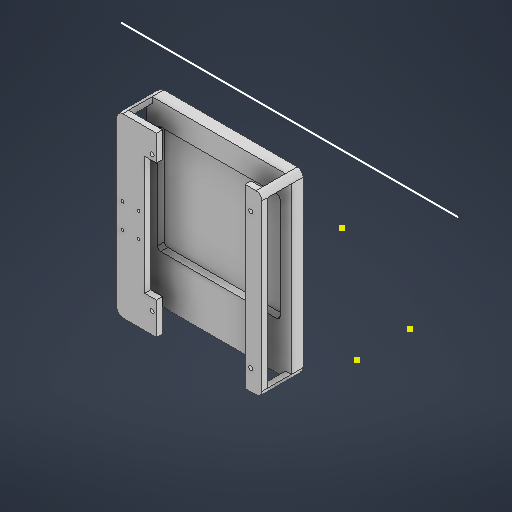
# Autodesk Inventor part: Box2
Saved by Autodesk Inventor 2026 (Build 300175000, 175)
## iProperties
Created: 2025-12-06
Part Number: Box2
Material: Generic
Document SubType Name: Modeling
Designer: sudis
Density: 1 g/cm^3
Appearance: Default
Author: sudis
Autodesk Inventor part; units mm, degrees
ref_plane "Work Plane1" through (-141.8656, 16.9601, -97.2578) normal (0, 0, -1) x (-1, 0, 0)
sketch "Sketch1" plane through (-141.8656, 16.9601, -97.2578) normal (0, 0, -1) x (-1, 0, 0)
  line L0 (61.5, 85.55) -> (-61.5, 85.55)
  line L1 (-61.5, 85.55) -> (-61.5, -85.55)
  line L2 (-61.5, -85.55) -> (61.5, -85.55)
  line L3 (61.5, -85.55) -> (61.5, 85.55)
  line L4 (-49.2, 45.05) -> (49.2, 45.05) projected
  arc A0 (-49.2, 45.25) -> (-51.5, 42.95) centre (-49.2, 42.95) ccw projected
  line L5 (-51.5, -42.95) -> (-51.5, 42.95) projected
  arc A1 (-51.5, -42.95) -> (-49.2, -45.25) centre (-49.2, -42.95) ccw projected
  line L6 (49.2, -45.25) -> (-49.2, -45.25) projected
  arc A2 (49.2, -45.25) -> (51.5, -42.95) centre (49.2, -42.95) ccw projected
  line L7 (51.5, 42.95) -> (51.5, -42.95) projected
  arc A3 (51.5, 42.95) -> (49.2, 45.25) centre (49.2, 42.95) ccw projected
  line L8 (-49.2, 45.25) -> (49.2, 45.25) projected
  line L9 (-1.4388, 35.9111) -> (-1.4388, 43.9889) projected
  ellipse E0 centre (-1.2387, 43.9887) end of major axis (-1.3802, 44.1302) minor radius 0.2 (-1.2389, 44.1888) -> (-1.4388, 43.9889) ccw projected
  line L10 (1.2389, 44.1888) -> (-1.2389, 44.1888) projected
  ellipse E1 centre (1.2387, 43.9887) end of major axis (1.3802, 44.1302) minor radius 0.2 (1.4388, 43.9889) -> (1.2389, 44.1888) ccw projected
  line L11 (1.4388, 43.9889) -> (1.4388, 35.9111) projected
  ellipse E2 centre (1.0386, 35.9114) end of major axis (1.3217, 35.6283) minor radius 0.4 (1.0389, 35.5112) -> (1.4388, 35.9111) ccw projected
  line L12 (-1.0389, 35.5112) -> (1.0389, 35.5112) projected
  ellipse E3 centre (-1.0386, 35.9114) end of major axis (-1.3217, 35.6283) minor radius 0.4 (-1.4388, 35.9111) -> (-1.0389, 35.5112) ccw projected
  arc A4 (1.3, 34.75) -> (1.9, 35.35) centre (1.3, 35.35) ccw projected
  line L13 (1.9, 40.81) -> (1.9, 35.35) projected
  arc A5 (2.1, 41.01) -> (1.9, 40.81) centre (2.1, 40.81) ccw projected
  line L14 (2.1, 41.01) -> (2.9, 41.01) projected
  arc A6 (2.9, 41.01) -> (2.9, 41.95) centre (2.9, 41.48) ccw projected
  line L15 (2.9, 41.95) -> (2.1, 41.95) projected
  arc A7 (1.9, 42.15) -> (2.1, 41.95) centre (2.1, 42.15) ccw projected
  line L16 (1.9, 43.9887) -> (1.9, 42.15) projected
  ellipse E4 centre (2.1, 43.9887) end of major axis (2.1, 44.1888) minor radius 0.2 (2.1, 44.1888) -> (1.9, 43.9887) ccw projected
  line L17 (48.7, 44.1888) -> (2.1, 44.1888) projected
  ellipse E5 centre (48.7, 43.1884) end of major axis (48.7, 44.1888) minor radius 1 (49.7, 43.1884) -> (48.7, 44.1888) ccw projected
  line L18 (49.7, 43.1884) -> (49.7, 39.02) projected
  arc A8 (49.5, 38.82) -> (49.7, 39.02) centre (49.5, 39.02) ccw projected
  line L19 (49.5, 38.82) -> (49.3, 38.82) projected
  arc A9 (49.3, 38.82) -> (49.3, 37.88) centre (49.3, 38.35) ccw projected
  line L20 (49.3, 37.88) -> (49.5, 37.88) projected
  arc A10 (49.7, 37.68) -> (49.5, 37.88) centre (49.5, 37.68) ccw projected
  line L21 (49.7, 37.68) -> (49.7, 33.65) projected
  arc A11 (48.7, 32.65) -> (49.7, 33.65) centre (48.7, 33.65) ccw projected
  line L22 (44.3574, 32.65) -> (48.7, 32.65) projected
  line L23 (44.3574, 32.65) -> (44.3574, 31.25) projected
  arc A12 (44.3574, 31.25) -> (46, 29.6074) centre (46, 31.25) ccw projected
  line L24 (46, 29.6074) -> (49.0579, 29.6074) projected
  spline S0 degree 3 poles (49.0579, 29.6074) (49.1602, 29.6074) (49.2528, 29.5891) (49.3382, 29.5567) (49.4237, 29.5242) (49.5019, 29.4774) (49.5659, 29.4253) (49.63, 29.3732) (49.6799, 29.3158) (49.7211, 29.2545) (49.7623, 29.1932) (49.7948, 29.128) (49.8186, 29.0541) (49.8423, 28.9803) (49.8574, 28.8977) (49.8574, 28.8079) knots 0.000001 0.000001 0.000001 0.000001 0.2 0.2 0.2 0.4 0.4 0.4 0.6 0.6 0.6 0.8 0.8 0.8 1 1 1 1 projected
  line L25 (49.8574, 28.8079) -> (49.8574, -24.3079) projected
  spline S1 degree 3 poles (49.8574, -24.3079) (49.8574, -24.3965) (49.8435, -24.4795) (49.8172, -24.5583) (49.7909, -24.6372) (49.7523, -24.712) (49.7048, -24.7778) (49.6573, -24.8437) (49.601, -24.9008) (49.5354, -24.9492) (49.4699, -24.9976) (49.3952, -25.0375) (49.3152, -25.0649) (49.2351, -25.0923) (49.1498, -25.1074) (49.0579, -25.1074) knots 0 0 0 0 0.2 0.2 0.2 0.4 0.4 0.4 0.6 0.6 0.6 0.8 0.8 0.8 1 1 1 1 projected
  line L26 (49.0579, -25.1074) -> (46, -25.1074) projected
  arc A13 (46, -25.1074) -> (46, -28.3926) centre (46, -26.75) ccw projected
  line L27 (46, -28.3926) -> (49.0579, -28.3926) projected
  spline S2 degree 3 poles (49.0579, -28.3926) (49.1602, -28.3926) (49.2528, -28.4109) (49.3382, -28.4433) (49.4237, -28.4758) (49.5019, -28.5226) (49.5659, -28.5747) (49.63, -28.6268) (49.6799, -28.6842) (49.7211, -28.7455) (49.7623, -28.8068) (49.7948, -28.872) (49.8186, -28.9459) (49.8423, -29.0197) (49.8574, -29.1023) (49.8574, -29.1921) knots 0.000001 0.000001 0.000001 0.000001 0.2 0.2 0.2 0.4 0.4 0.4 0.6 0.6 0.6 0.8 0.8 0.8 1 1 1 1 projected
  line L28 (49.8574, -29.1921) -> (49.8574, -42.95) projected
  arc A14 (49.2, -43.6074) -> (49.8574, -42.95) centre (49.2, -42.95) ccw projected
  line L29 (49.2, -43.6074) -> (-49.2, -43.6074) projected
  arc A15 (-49.8574, -42.95) -> (-49.2, -43.6074) centre (-49.2, -42.95) ccw projected
  line L30 (-49.8574, -42.95) -> (-49.8574, -29.1921) projected
  spline S3 degree 3 poles (-49.8574, -29.1921) (-49.8574, -29.1035) (-49.8435, -29.0205) (-49.8172, -28.9417) (-49.7909, -28.8628) (-49.7523, -28.788) (-49.7048, -28.7222) (-49.6573, -28.6563) (-49.601, -28.5992) (-49.5354, -28.5508) (-49.4699, -28.5024) (-49.3952, -28.4625) (-49.3152, -28.4351) (-49.2351, -28.4077) (-49.1498, -28.3926) (-49.0579, -28.3926) knots 0 0 0 0 0.2 0.2 0.2 0.4 0.4 0.4 0.6 0.6 0.6 0.8 0.8 0.8 1 1 1 1 projected
  line L31 (-49.0579, -28.3926) -> (-40, -28.3926) projected
  arc A16 (-40, -28.3926) -> (-40, -25.1074) centre (-40, -26.75) ccw projected
  line L32 (-40, -25.1074) -> (-49.0579, -25.1074) projected
  spline S4 degree 3 poles (-49.0579, -25.1074) (-49.1602, -25.1074) (-49.2528, -25.0891) (-49.3382, -25.0567) (-49.4237, -25.0242) (-49.5019, -24.9774) (-49.5659, -24.9253) (-49.63, -24.8732) (-49.6799, -24.8158) (-49.7211, -24.7545) (-49.7623, -24.6932) (-49.7948, -24.628) (-49.8186, -24.5541) (-49.8423, -24.4803) (-49.8574, -24.3977) (-49.8574, -24.3079) knots 0.000001 0.000001 0.000001 0.000001 0.2 0.2 0.2 0.4 0.4 0.4 0.6 0.6 0.6 0.8 0.8 0.8 1 1 1 1 projected
  line L33 (-49.8574, -24.3079) -> (-49.8574, 25.9079) projected
  spline S5 degree 3 poles (-49.8574, 25.9079) (-49.8574, 26.0102) (-49.8391, 26.1028) (-49.8067, 26.1882) (-49.7742, 26.2737) (-49.7274, 26.3519) (-49.6753, 26.4159) (-49.6232, 26.48) (-49.5658, 26.5299) (-49.5045, 26.5711) (-49.4432, 26.6123) (-49.378, 26.6448) (-49.3041, 26.6686) (-49.2303, 26.6923) (-49.1477, 26.7074) (-49.0579, 26.7074) knots 0.000001 0.000001 0.000001 0.000001 0.2 0.2 0.2 0.4 0.4 0.4 0.6 0.6 0.6 0.8 0.8 0.8 1 1 1 1 projected
  line L34 (-49.0579, 26.7074) -> (-36.4, 26.7074) projected
  arc A17 (-36.4, 26.7074) -> (-34.3574, 28.75) centre (-36.4, 28.75) ccw projected
  line L35 (-34.3574, 28.75) -> (-34.3574, 32.65) projected
  line L36 (-34.3574, 32.65) -> (-48.7, 32.65) projected
  arc A18 (-49.7, 33.65) -> (-48.7, 32.65) centre (-48.7, 33.65) ccw projected
  line L37 (-49.7, 33.65) -> (-49.7, 37.68) projected
  arc A19 (-49.5, 37.88) -> (-49.7, 37.68) centre (-49.5, 37.68) ccw projected
  line L38 (-49.5, 37.88) -> (-49.3, 37.88) projected
  arc A20 (-49.3, 37.88) -> (-49.3, 38.82) centre (-49.3, 38.35) ccw projected
  line L39 (-49.3, 38.82) -> (-49.5, 38.82) projected
  arc A21 (-49.7, 39.02) -> (-49.5, 38.82) centre (-49.5, 39.02) ccw projected
  line L40 (-49.7, 39.02) -> (-49.7, 43.1884) projected
  ellipse E6 centre (-48.7, 43.1884) end of major axis (-48.7, 44.1888) minor radius 1 (-48.7, 44.1888) -> (-49.7, 43.1884) ccw projected
  line L41 (-2.1, 44.1888) -> (-48.7, 44.1888) projected
  ellipse E7 centre (-2.1, 43.9887) end of major axis (-2.1, 44.1888) minor radius 0.2 (-1.9, 43.9887) -> (-2.1, 44.1888) ccw projected
  line L42 (-1.9, 35.69) -> (-1.9, 43.9887) projected
  line L43 (-1.9, 35.69) -> (-2.9, 35.69) projected
  arc A22 (-2.9, 35.69) -> (-2.9, 34.75) centre (-2.9, 35.22) ccw projected
  line L44 (-2.9, 34.75) -> (1.3, 34.75) projected
  line L45 (36.45, -75.55) -> (36.45, 75.55) projected
  line L46 (-36.45, -75.55) -> (36.45, -75.55) projected
  line L47 (-36.45, 75.55) -> (-36.45, -75.55) projected
  line L48 (36.45, 75.55) -> (-36.45, 75.55) projected
  point P0 (-141.8656, -16.9601)
  dimension "d2" = 10
  dimension "d3" = 10
  dimension "d4" = 10
  dimension "d5" = 10
  constraints: 8 end point, 2 parallel, 1 horizontal, 1 perpendicular, 8 other
  measures "d2" distance between parallel lines of L48 L0
  measures "d3" distance between parallel lines of L2 L46
  measures "d4" distance between parallel lines of L1 L5
  measures "d5" distance between parallel lines of L3 L7
extrude "Extrusion1" add sketch "Sketch1" against normal blind 85 contours L3 L2 L1 L0 | L47 L8 L45 L4 | L47 L41 E6 L40 A21 L39 A20 L38 A19 L37 A18 L36 L34 S5 L33 S4 L32 A16 L31 S3 L30 A15 L29 L6 A1 L5 A0 L8 | L4 L45 L17 E4 L16 A7 L15 A6 L14 A5 L13 A4 L44 A22 L43 L42 E7 L41 L47 | L45 L8 A3 L7 A2 L6 L29 A14 L28 S2 L27 A13 L26 S1 L25 S0 L24 A12 L23 L22 A11 L21 A10 L20 A9 L19 A8 L18 E5 L17 | L47 L48 L45 L8 | L47 L36 A18 L37 A19 L38 A20 L39 A21 L40 E6 L41 | L41 E7 L42 L43 A22 L44 A4 L13 A5 L14 A6 L15 A7 L16 E4 L17 L45 L29 L47 L34 A17 L35 L36 | L17 E5 L18 A8 L19 A9 L20 A10 L21 A11 L22 L23 A12 L24 S0 L25 S1 L26 A13 L27 S2 L28 A14 L29 L45 | L36 L35 A17 L34 L47 | L45 L6 L47 L29 | L47 L29 A15 L30 S3 L31 A16 L32 S4 L33 S5 L34 | L45 L46 L47 L6 | L9 E0 L10 E1 L11 E2 L12 E3
sketch "Sketch2" plane through (-80.3656, -68.5899, -97.2578) normal (1, 0, 0) x (0, 0, -1)
  line L0 (-80, 5) -> (-5, 5)
  line L1 (-5, 5) -> (-5, 166.1)
  line L2 (-5, 166.1) -> (-80, 166.1)
  line L3 (-80, 166.1) -> (-80, 5)
  line L4 (-85, 0) -> (-85, 171.1) projected
  line L5 (0, 171.1) -> (-85, 171.1) projected
  line L6 (0, 171.1) -> (0, 0) projected
  line L7 (0, 0) -> (-85, 0) projected
  point P0 (-97.2578, 68.5899)
  point P1 (-42.5, 171.1)
  dimension "d8" = 5
  dimension "d9" = 5
  dimension "d10" = 5
  dimension "d11" = 5
  constraints: 8 end point, 2 parallel, 1 horizontal, 1 midpoint, 1 perpendicular
  measures "d8" distance between parallel lines of L4 L3
  measures "d9" distance from line of point (-42.5, 171.1) L2
  measures "d10" distance between parallel lines of L6 L1
  measures "d11" distance between parallel lines of L7 L0
extrude "Extrusion2" cut sketch "Sketch2" against normal blind 237.5 contours L3 L2 L1 L0
sketch "Sketch3" plane through (-203.3656, -68.5899, -97.2578) normal (0, -1, 0) x (1, 0, 0)
  line L0 (5, 80) -> (118, 80)
  line L1 (118, 80) -> (118, 5)
  line L2 (118, 5) -> (5, 5)
  line L3 (5, 5) -> (5, 80)
  line L4 (0, 85) -> (123, 85) projected
  line L5 (123, 0) -> (123, 85) projected
  line L6 (123, 0) -> (0, 0) projected
  line L7 (0, 0) -> (0, 85) projected
  point P0 (203.3656, 97.2578)
  dimension "d14" = 5
  dimension "d15" = 5
  dimension "d16" = 5
  dimension "d17" = 5
  constraints: 8 end point, 2 parallel, 1 horizontal, 1 perpendicular
  measures "d14" distance between parallel lines of L4 L0
  measures "d15" distance between parallel lines of L5 L1
  measures "d16" distance between parallel lines of L6 L2
  measures "d17" distance between parallel lines of L7 L3
extrude "Extrusion3" cut sketch "Sketch3" against normal blind 402.2625 contours L0 L1 L2 L3
sketch "Sketch4" plane through (-80.3656, -63.5899, -92.2578) normal (0, 0, 1) x (1, 0, 0)
  line L0 (-97.95, 5) -> (-97.95, 156.1) projected
  line L1 (-25.05, 5) -> (-97.95, 5) projected
  line L2 (-25.05, 156.1) -> (-25.05, 5) projected
  line L3 (-97.95, 156.1) -> (-25.05, 156.1) projected
  line L4 (-98.2, 156.35) -> (-98.2, 4.75)
  line L5 (-98.2, 4.75) -> (-24.8, 4.75)
  line L6 (-24.8, 4.75) -> (-24.8, 156.35)
  line L7 (-24.8, 156.35) -> (-98.2, 156.35)
  point P0 (80.3656, 63.5899)
  dimension "d20" = 0.25
  constraints: 8 end point, 3 other
  measures "d20" distance between parallel lines of L0 L4
sketch "Sketch5" plane through (-141.8656, 16.9601, -97.2578) normal (0, 0, -1) x (-1, 0, 0)
  line L0 (-61.5, 85.55) -> (-61.5, -85.55) projected
  line L1 (-61.5, -85.55) -> (61.5, -85.55) projected
  line L2 (61.5, -85.55) -> (61.5, 85.55) projected
  line L3 (61.5, 85.55) -> (-61.5, 85.55) projected
  point P0 (-141.8656, -16.9601)
extrude "Extrusion4" add sketch "Sketch5" along normal blind 5
extrude "Extrusion5" cut sketch "Sketch4" against normal blind 7 contours L0 L3 L2 L1 | L7 L6 L5 L4
sketch "Sketch6" plane through (-203.3656, 102.5101, -12.2578) normal (0, 1, 0) x (1, 0, 0)
  line L0 (-40.6731, 44.9) -> (244.0387, 44.9)
  point P0 (203.3656, -12.2578)
  constraints: 2 end point, 1 horizontal, 2 other
sketch "Sketch7" plane through (-203.3656, 102.5101, -12.2578) normal (0, 1, 0) x (1, 0, 0)
  line L0 (118, 80) -> (118, 5) projected
  line L1 (118, 44.9) -> (5, 44.9)
  line L2 (5, 44.9) -> (5, 54.9)
  line L3 (5, 54.9) -> (118, 54.9)
  line L4 (118, 54.9) -> (118, 44.9)
  line L5 (-40.6731, 44.9) -> (244.0387, 44.9) projected
  line L6 (5, 5) -> (5, 80) projected
  point P0 (203.3656, -12.2578)
  dimension "d25" = 0
  dimension "d26" = 0
  dimension "d27" = 10
  constraints: 8 end point, 2 parallel, 1 horizontal, 1 perpendicular, 1 point on line
  measures "d25" distance between parallel lines of L1 L5
  measures "d26" distance between parallel lines of L6 L2
  measures "d27" distance between parallel lines of L1 L3
extrude "Extrusion6" add sketch "Sketch7" against normal up to surface (171.1 mm away)
sketch "Sketch8" plane through (-198.3656, 102.5101, -57.1578) normal (0, 0, 1) x (1, 0, 0)
  point P0 (198.3656, -102.5101)
sketch "Sketch9" plane through (-198.3656, 102.5101, -57.1578) normal (0, 0, 1) x (1, 0, 0)
  arc A0 (7.3, -40.3) -> (5, -42.6) centre (7.3, -42.6) ccw projected
  line L0 (105.7, -40.3) -> (7.3, -40.3) projected
  line L1 (5, -42.6) -> (5, -128.5) projected
  arc A1 (5, -128.5) -> (7.3, -130.8) centre (7.3, -128.5) ccw projected
  line L2 (7.3, -130.8) -> (105.7, -130.8) projected
  line L3 (108, -128.5) -> (108, -42.6) projected
  arc A2 (105.7, -130.8) -> (108, -128.5) centre (105.7, -128.5) ccw projected
  arc A3 (108, -42.6) -> (105.7, -40.3) centre (105.7, -42.6) ccw projected
  line L4 (105.7, -131.05) -> (7.3, -131.05)
  arc A4 (4.75, -128.5) -> (7.3, -131.05) centre (7.3, -128.5) ccw
  line L5 (4.75, -128.5) -> (4.75, -42.6)
  arc A5 (7.3, -40.05) -> (4.75, -42.6) centre (7.3, -42.6) ccw
  line L6 (7.3, -40.05) -> (105.7, -40.05)
  arc A6 (108.25, -42.6) -> (105.7, -40.05) centre (105.7, -42.6) ccw
  line L7 (108.25, -42.6) -> (108.25, -128.5)
  arc A7 (105.7, -131.05) -> (108.25, -128.5) centre (105.7, -128.5) ccw
  point P0 (198.3656, -102.5101)
  dimension "d30" = 0.25
  constraints: 8 end point, 8 point on circle, 4 centre point, 7 other
  measures "d30" distance between parallel lines of L2 L4
extrude "Extrusion7" cut sketch "Sketch9" against normal blind 7.25 contours L0 A3 L3 A2 L2 A1 L1 A0 | L4 A4 L5 A5 L6 A6 L7 A7
sketch "Sketch10" plane through (-80.3656, -68.5899, -12.2578) normal (1, 0, 0) x (0, 0, -1)
  line L0 (54.9, 166.1) -> (54.9, 5) projected
  line L1 (80, 5) -> (5, 5) projected
  line L2 (80, 166.1) -> (80, 5) projected
  line L3 (5, 166.1) -> (80, 166.1) projected
  point P0 (-12.2578, 68.5899)
extrude "Extrusion8" add sketch "Sketch10" against normal up to surface (5 mm away)
ref_plane "Work Plane2" through (-141.8656, -68.5899, -12.2578) normal (-1, 0, 0) x (0, 0, 1)
mirror "Mirror1" about plane through (-141.8656, -68.5899, -12.2578) normal (-1, 0, 0) of "Extrusion8"
sketch "Sketch11" plane through (-203.3656, -68.5899, -12.2578) normal (0, -1, 0) x (1, 0, 0)
  line L0 (118, -54.9) -> (5, -54.9) projected
  line L1 (5, -80) -> (5, -54.9) projected
  line L2 (118, -80) -> (5, -80) projected
  line L3 (118, -54.9) -> (118, -80) projected
  point P0 (203.3656, 12.2578)
extrude "Extrusion9" add sketch "Sketch11" against normal blind 2.5
sketch "Sketch12" plane through (-85.3656, -63.5899, -57.1578) normal (1, 0, 0) x (0, 0, -1)
  line L0 (10, 0) -> (0, 0) projected
  line L1 (10, 161.1) -> (10, 0) projected
  line L2 (0, 161.1) -> (10, 161.1) projected
  line L3 (0, 161.1) -> (0, 0) projected
  point P0 (-57.1578, 63.5899)
extrude "Extrusion10" add sketch "Sketch12" along normal up to surface (5 mm away)
mirror "Mirror2" about plane through (-141.8656, -68.5899, -12.2578) normal (-1, 0, 0) of "Extrusion10"
sketch "Sketch13" plane through (-141.8656, 16.9601, -12.2578) normal (0, 0, 1) x (1, 0, 0)
  point P0 (141.8656, -16.9601)
sketch "Sketch14" plane through (-141.8656, 16.9601, -12.2578) normal (0, 0, 1) x (1, 0, 0)
  line L0 (-36.45, -75.55) -> (-36.45, 75.55) projected
  line L1 (36.45, -75.55) -> (-36.45, -75.55) projected
  line L2 (36.45, 75.55) -> (36.45, -75.55) projected
  line L3 (-36.45, 75.55) -> (36.45, 75.55) projected
  arc A0 (-51.3, -42.95) -> (-49.2, -45.05) centre (-49.2, -42.95) ccw projected
  line L4 (-49.2, -45.05) -> (49.2, -45.05) projected
  arc A1 (49.2, -45.05) -> (51.3, -42.95) centre (49.2, -42.95) ccw projected
  line L5 (51.3, -42.95) -> (51.3, 42.95) projected
  arc A2 (51.3, 42.95) -> (49.2, 45.05) centre (49.2, 42.95) ccw projected
  line L6 (49.2, 45.05) -> (-49.2, 45.05) projected
  arc A3 (-49.2, 45.05) -> (-51.3, 42.95) centre (-49.2, 42.95) ccw projected
  line L7 (-51.3, 42.95) -> (-51.3, -42.95) projected
  arc A4 (50.2559, 34.65) -> (49.4, 35.5059) centre (49.4, 34.65) ccw projected
  line L8 (50.2559, -43.15) -> (50.2559, 34.65) projected
  arc A5 (49.4, -44.0059) -> (50.2559, -43.15) centre (49.4, -43.15) ccw projected
  line L9 (-49.4, -44.0059) -> (49.4, -44.0059) projected
  arc A6 (-50.2559, -43.15) -> (-49.4, -44.0059) centre (-49.4, -43.15) ccw projected
  line L10 (-50.2559, 34.65) -> (-50.2559, -43.15) projected
  arc A7 (-49.4, 35.5059) -> (-50.2559, 34.65) centre (-49.4, 34.65) ccw projected
  line L11 (49.4, 35.5059) -> (-49.4, 35.5059) projected
  line L12 (-56.5, 46.1504) -> (56.5, 46.1504)
  line L13 (56.5, 46.1504) -> (56.5, 80.55)
  line L14 (56.5, 80.55) -> (-56.5, 80.55)
  line L15 (-56.5, 80.55) -> (-56.5, 46.1504)
  line L16 (-61.5, 85.55) -> (-61.5, -85.55) projected
  line L17 (61.5, -85.55) -> (61.5, 85.55) projected
  line L18 (61.5, 85.55) -> (-61.5, 85.55) projected
  point P0 (141.8656, -16.9601)
  point P1 (56.5, 63.3502)
  dimension "d39" = 5
  dimension "d40" = 5
  dimension "d41" = 5
  constraints: 8 end point, 2 parallel, 1 horizontal, 1 midpoint, 1 perpendicular
  measures "d39" distance between parallel lines of L16 L15
  measures "d40" distance from line of L17 point (56.5, 63.35)
  measures "d41" distance between parallel lines of L18 L14
extrude "Extrusion11" cut sketch "Sketch14" against normal blind 69.375 contours L12 L15 L14 L13 L2 L3 L0 | L0 L3 L2 L12
sketch "Sketch15" plane through (-141.8656, 16.9601, -12.2578) normal (0, 0, 1) x (1, 0, 0)
  circle A0 centre (-42.5, -9.2) radius 1.2 projected
  circle A1 centre (-56, -9.2) radius 1.2 projected
  circle A2 centre (-56, -30.2) radius 1.2 projected
  circle A3 centre (-42.5, -30.2) radius 1.2 projected
  circle A4 centre (-35, 36.8) radius 2.7813 projected
  circle A5 centre (52, 36.8) radius 2.7813 projected
  circle A6 centre (-35, -76.2) radius 2.7813 projected
  circle A7 centre (52, -76.2) radius 2.7813 projected
  point P0 (141.8656, -16.9601)
hole "Hole1" at (-176.8656, 53.7601, -12.2578) at (-176.8656, -59.2399, -12.2578) at (-89.8656, -59.2399, -12.2578) at (-89.8656, 53.7601, -12.2578) direction (0, 0, -1) diameter 3.4 depth 5 clearance for "Flat Head Machine Screw" size "M3" standard "Ansi Metric M Profile"
sketch "Sketch16" plane through (-141.8656, 16.9601, -12.2578) normal (0, 0, 1) x (1, 0, 0)
  circle A0 centre (-42.5, -9.2) radius 1.2 projected
  circle A1 centre (-56, -9.2) radius 1.2 projected
  circle A2 centre (-56, -30.2) radius 1.2 projected
  circle A3 centre (-42.5, -30.2) radius 1.2 projected
  point P0 (141.8656, -16.9601)
hole "Hole2" at (-184.3656, 7.7601, -12.2578) at (-197.8656, 7.7601, -12.2578) at (-197.8656, -13.2399, -12.2578) at (-184.3656, -13.2399, -12.2578) direction (0, 0, -1) diameter 2.4 depth 5 clearance for "Flat Head Machine Screw" size "M2" standard "Ansi Metric M Profile"
sketch "Sketch17" plane through (-141.8656, 16.9601, -102.2578) normal (0, 0, -1) x (-1, 0, 0)
  line L0 (-61.5, -85.55) -> (61.5, -85.55) projected
  line L1 (61.5, -85.55) -> (61.5, 85.55) projected
  line L2 (61.5, 85.55) -> (-61.5, 85.55) projected
  line L3 (-61.5, 85.55) -> (-61.5, -85.55) projected
  point P0 (-141.8656, -16.9601)
extrude "Extrusion12" cut sketch "Sketch17" against normal up to surface (35.1 mm away)
sketch "Sketch18" plane through (-198.3656, -68.5899, -57.1578) normal (0, 0, 1) x (1, 0, 0)
  line L0 (113, 166.1) -> (113, 131.7004) construction
  line L1 (113, 131.7004) -> (0, 131.7004) construction
  line L2 (0, 166.1) -> (113, 166.1) construction
  line L3 (0, 131.7004) -> (0, 166.1) construction
  line L4 (0, 166.1) -> (113, 166.1) projected
  line L5 (113, 166.1) -> (113, 131.7004) projected
  line L6 (113, 131.7004) -> (0, 131.7004) projected
  line L7 (0, 131.7004) -> (0, 166.1) projected
  point P0 (198.3656, 68.5899)
extrude "Extrusion13" add sketch "Sketch18" against normal up to surface (10 mm away)
sketch "Sketch19" plane through (-141.8656, 16.9601, -12.2578) normal (0, 0, 1) x (1, 0, 0)
  line L0 (56.5, 46.1504) -> (-56.5, 46.1504) projected
  line L1 (56.5, 80.55) -> (56.5, 46.1504) projected
  line L2 (-56.5, 80.55) -> (56.5, 80.55) projected
  line L3 (-56.5, 46.1504) -> (-56.5, 80.55) projected
  point P0 (141.8656, -16.9601)
extrude "Extrusion14" add sketch "Sketch19" against normal up to surface (5 mm away)
sketch "Sketch20" plane through (-141.8656, 16.9601, -12.2578) normal (0, 0, 1) x (1, 0, 0)
  circle A0 centre (-42.5, -30.2) radius 1.2 projected
  circle A1 centre (-42.5, -9.2) radius 1.2 projected
  circle A2 centre (-42.5, -30.2) radius 1.2 projected
  circle A3 centre (-56, -30.2) radius 1.2 projected
  circle A4 centre (-56, -9.2) radius 1.2 projected
  circle A5 centre (-42.5, -9.2) radius 1.2 projected
  circle A6 centre (52, 36.8) radius 1.7 projected
  circle A7 centre (52, -76.2) radius 1.7 projected
  circle A8 centre (-35, -76.2) radius 1.7 projected
  circle A9 centre (-35, 36.8) radius 1.7 projected
  line L0 (61.5, -85.55) -> (61.5, 85.55) projected
  line L1 (61.5, 85.55) -> (-61.5, 85.55) projected
  line L2 (-61.5, 85.55) -> (-61.5, -85.55) projected
  line L3 (-61.5, -85.55) -> (61.5, -85.55) projected
  circle A10 centre (-35, -76.2) radius 1.7 projected
  circle A11 centre (-35, 36.8) radius 1.7 projected
  circle A12 centre (52, 36.8) radius 1.7 projected
  circle A13 centre (52, -76.2) radius 1.7 projected
  point P0 (141.8656, -16.9601)
extrude "Extrusion15" add sketch "Sketch20" against normal up to surface (5 mm away) contours A0 | A1 | A3 | A4 | A6 | A7 | A8 | A9
sketch "Sketch21" plane through (-141.8656, 16.9601, -12.2578) normal (0, 0, 1) x (1, 0, 0)
  line L0 (-61.5, 85.55) -> (-61.5, -85.55) projected
  line L1 (61.5, -85.55) -> (61.5, 85.55) projected
  line L2 (-61.5, -85.55) -> (61.5, -85.55) projected
  line L3 (61.5, 85.55) -> (-61.5, 85.55) projected
  line L4 (56.5, 85.55) -> (-56.5, 85.55) projected
  point P0 (141.8656, -16.9601)
  point P1 (52, -68.138)
  point P2 (52, 46.862)
  point P3 (-31.5, 46.862)
  point P4 (-31.5, -68.138)
  point P5 (-43, -21.138)
  point P6 (-43, -0.138)
  point P7 (-56.5, -21.138)
  point P8 (-56.5, -0.138)
  dimension "d76" = 17.412
  dimension "d78" = 30
  dimension "d80" = 30
  dimension "d81" = 83.5
  dimension "d82" = 83.5
  dimension "d83" = 13.5
  dimension "d84" = 13.5
  dimension "d85" = 21
  dimension "d87" = 5
  dimension "d129" = 64.412
  dimension "d131" = 115
  dimension "d132" = 17.412
  dimension "d133" = 115
  measures "d76" distance from line of L2 point (52, -68.138)
  measures "d78" distance from line of point (-31.5, -68.138) L0
  measures "d80" distance from line of L0 point (-31.5, 46.862)
  measures "d81" distance of point (52, -68.138) point (-31.5, -68.138)
  measures "d82" distance of point (52, 46.862) point (-31.5, 46.862)
  measures "d83" distance of point (-43, -21.138) point (-56.5, -21.138)
  measures "d84" distance of point (-43, -0.138) point (-56.5, -0.138)
  measures "d85" distance of point (-56.5, -0.138) point (-56.5, -21.138)
  measures "d87" distance from line of L0 point (-56.5, -0.138)
  measures "d129" distance from line of L2 point (-56.5, -21.138)
  measures "d131" distance of point (52, 46.862) point (52, -68.138)
  measures "d132" distance from line of L2 point (-31.5, -68.138)
  measures "d133" distance of point (-31.5, -68.138) point (-31.5, 46.862)
sketch "Sketch22" plane through (-141.8656, 16.9601, -12.2578) normal (0, 0, 1) x (1, 0, 0)
  line L0 (61.5, -85.55) -> (61.5, 85.55) projected
  line L1 (61.5, 85.55) -> (-61.5, 85.55) projected
  line L2 (-61.5, 85.55) -> (-61.5, -85.55) projected
  line L3 (-61.5, -85.55) -> (61.5, -85.55) projected
  line L4 (61.5, 85.55) -> (-61.5, 85.55)
  line L5 (-61.5, 85.55) -> (-61.5, 64.2739)
  line L6 (-61.5, 64.2739) -> (61.5, 64.2739)
  line L7 (61.5, 64.2739) -> (61.5, 85.55)
  point P0 (141.8656, -16.9601)
  point P1 (61.5, 64.2739)
  constraints: 8 end point, 2 parallel, 1 horizontal, 1 perpendicular, 1 point on line
extrude "Extrusion16" cut sketch "Sketch22" against normal blind 79.85 contours L6 L2 L1 L0
sketch "Sketch23" plane through (-141.8656, 16.9601, -12.2578) normal (0, 0, 1) x (1, 0, 0)
  line L0 (61.5, 64.2739) -> (-61.5, 64.2739) projected
  line L1 (-27.7565, 64.2739) -> (47.2435, 64.2739)
  line L2 (47.2435, 64.2739) -> (47.2435, 14.2739)
  line L3 (47.2435, 14.2739) -> (-27.7565, 14.2739)
  line L4 (-27.7565, 14.2739) -> (-27.7565, 64.2739)
  point P0 (141.8656, -16.9601)
  point P1 (47.2435, 64.2739)
  dimension "d108" = 50
  dimension "d109" = 75
  constraints: 8 end point, 2 parallel, 1 horizontal, 1 perpendicular, 1 point on line
  measures "d108" distance of L1.end L2.end
  measures "d109" distance of L2.end L3.end
extrude "Extrusion17" cut sketch "Sketch23" against normal up to surface (5 mm away)
sketch "Sketch24" plane through (-85.3656, -68.5899, -17.2578) normal (0, 0, -1) x (-1, 0, 0)
  line L0 (84.2565, 149.8239) -> (84.2565, 99.8239) projected
  line L1 (84.2565, 99.8239) -> (9.2565, 99.8239) projected
  line L2 (9.2565, 99.8239) -> (9.2565, 149.8239) projected
  line L3 (9.2565, 149.8239) -> (-5, 149.8239) projected
  line L4 (-5, 5) -> (-5, 149.8239) projected
  line L5 (-5, 5) -> (0, 5) projected
  line L6 (0, 0) -> (0, 5) projected
  line L7 (113, 0) -> (0, 0) projected
  line L8 (113, 0) -> (113, 5) projected
  line L9 (113, 5) -> (118, 5) projected
  line L10 (118, 149.8239) -> (118, 5) projected
  line L11 (118, 149.8239) -> (84.2565, 149.8239) projected
  point P0 (-85.3656, 68.5899)
sketch "Sketch25" plane through (-198.3656, -68.5899, -57.1578) normal (0, 0, 1) x (1, 0, 0)
  line L0 (118, 149.8239) -> (-5, 149.8239) projected
  line L1 (-5, 5) -> (-5, 149.8239) projected
  line L2 (0, 5) -> (-5, 5) projected
  line L3 (0, 0) -> (0, 5) projected
  line L4 (0, 0) -> (113, 0) projected
  line L5 (113, 5) -> (113, 0) projected
  line L6 (118, 5) -> (113, 5) projected
  line L7 (118, 5) -> (118, 149.8239) projected
  arc A0 (7.3, 131.05) -> (4.75, 128.5) centre (7.3, 128.5) ccw projected
  line L8 (7.3, 131.05) -> (105.7, 131.05) projected
  arc A1 (108.25, 128.5) -> (105.7, 131.05) centre (105.7, 128.5) ccw projected
  line L9 (108.25, 128.5) -> (108.25, 42.6) projected
  arc A2 (105.7, 40.05) -> (108.25, 42.6) centre (105.7, 42.6) ccw projected
  line L10 (105.7, 40.05) -> (7.3, 40.05) projected
  arc A3 (4.75, 42.6) -> (7.3, 40.05) centre (7.3, 42.6) ccw projected
  line L11 (4.75, 42.6) -> (4.75, 128.5) projected
  line L12 (118, 149.8239) -> (113, 149.8239)
  line L13 (113, 149.8239) -> (113, 144.8239)
  line L14 (113, 144.8239) -> (118, 144.8239)
  line L15 (118, 144.8239) -> (118, 149.8239)
  line L16 (-5, 149.8239) -> (0, 149.8239)
  line L17 (0, 149.8239) -> (0, 144.8239)
  line L18 (0, 144.8239) -> (-5, 144.8239)
  line L19 (-5, 144.8239) -> (-5, 149.8239)
  point P0 (198.3656, 68.5899)
  point P1 (118, 144.8239)
  point P2 (113, 149.8239)
  dimension "d112" = 5
  dimension "d113" = 5
  dimension "d114" = 5
  dimension "d115" = 5
  constraints: 16 end point, 4 parallel, 2 horizontal, 2 perpendicular
  measures "d112" distance of L14.end L13.end
  measures "d113" distance of L13.end L12.end
  measures "d114" distance of L17.end L18.end
  measures "d115" distance of L16.end L17.end
extrude "Extrusion18" add sketch "Sketch25" along normal up to surface (39.9 mm away) contours L7 L14 L13 L0 | L17 L18 L1 L0
sketch "Sketch26" plane through (-141.8656, 16.9601, -12.2578) normal (0, 0, 1) x (1, 0, 0)
  line L0 (47.2435, 14.2739) -> (-27.7565, 14.2739) projected
  line L1 (-27.7565, 14.2739) -> (-27.7565, -85.55)
  line L2 (-56.5, -85.55) -> (56.5, -85.55) projected
  line L3 (47.2435, 64.2739) -> (47.2435, 14.2739) projected
  line L4 (47.2435, 14.2739) -> (47.2435, -85.55)
  line L5 (-61.5, -85.55) -> (61.5, -85.55) projected
  point P0 (141.8656, -16.9601)
  constraints: 4 end point, 2 vertical, 1 point on line
extrude "Extrusion19" cut sketch "Sketch26" against normal up to surface (5 mm away)
ref_plane "Work Plane4" through (-198.3656, -68.5899, -37.2078) normal (0, 0, 1) x (1, 0, 0)
sketch "Sketch27" plane through (-198.3656, -68.5899, -37.2078) normal (0, 0, 1) x (1, 0, 0)
  line L0 (0, 144.8239) -> (-5, 144.8239) projected
  line L1 (-5, 5) -> (-5, 144.8239) projected
  line L2 (0, 5) -> (-5, 5) projected
  line L3 (0, 0) -> (0, 5) projected
  line L4 (0, 0) -> (113, 0) projected
  line L5 (113, 5) -> (113, 0) projected
  line L6 (118, 5) -> (113, 5) projected
  line L7 (118, 5) -> (118, 144.8239) projected
  line L8 (118, 144.8239) -> (113, 144.8239) projected
  line L9 (113, 144.8239) -> (113, 149.8239) projected
  line L10 (113, 149.8239) -> (0, 149.8239) projected
  line L11 (0, 149.8239) -> (0, 144.8239) projected
  arc A0 (7.3, 131.05) -> (4.75, 128.5) centre (7.3, 128.5) ccw projected
  line L12 (7.3, 131.05) -> (105.7, 131.05) projected
  arc A1 (108.25, 128.5) -> (105.7, 131.05) centre (105.7, 128.5) ccw projected
  line L13 (108.25, 128.5) -> (108.25, 42.6) projected
  arc A2 (105.7, 40.05) -> (108.25, 42.6) centre (105.7, 42.6) ccw projected
  line L14 (105.7, 40.05) -> (7.3, 40.05) projected
  arc A3 (4.75, 42.6) -> (7.3, 40.05) centre (7.3, 42.6) ccw projected
  line L15 (4.75, 42.6) -> (4.75, 128.5) projected
  point P0 (198.3656, 68.5899)
extrude "Extrusion20" add sketch "Sketch27" against normal blind 10
sketch "Sketch28" plane through (-198.3656, -68.5899, -47.2078) normal (0, 0, -1) x (-1, 0, 0)
  line L0 (-7.3, 40.05) -> (-105.7, 40.05) projected
  arc A0 (-108.25, 42.6) -> (-105.7, 40.05) centre (-105.7, 42.6) ccw projected
  line L1 (-108.25, 42.6) -> (-108.25, 128.5) projected
  arc A1 (-105.7, 131.05) -> (-108.25, 128.5) centre (-105.7, 128.5) ccw projected
  line L2 (-105.7, 131.05) -> (-7.3, 131.05) projected
  arc A2 (-4.75, 128.5) -> (-7.3, 131.05) centre (-7.3, 128.5) ccw projected
  line L3 (-4.75, 128.5) -> (-4.75, 42.6) projected
  arc A3 (-7.3, 40.05) -> (-4.75, 42.6) centre (-7.3, 42.6) ccw projected
  point P0 (-198.3656, 68.5899)
extrude "Extrusion21" add sketch "Sketch28" against normal blind 4
sketch "Sketch29" plane through (-80.3656, -68.5899, -67.1578) normal (0, 0, -1) x (-1, 0, 0)
  line L0 (123, 149.8239) -> (0, 149.8239) projected
  line L1 (0, 0) -> (0, 149.8239) projected
  line L2 (123, 0) -> (0, 0) projected
  line L3 (123, 149.8239) -> (123, 0) projected
  point P0 (-80.3656, 68.5899)
extrude "Extrusion22" cut sketch "Sketch29" against normal up to surface (19.95 mm away)
sketch "Sketch30" plane through (-198.3656, -68.5899, -37.2078) normal (0, 0, 1) x (1, 0, 0)
  line L0 (7.3, 131.05) -> (105.7, 131.05) projected
  arc A0 (7.3, 131.05) -> (4.75, 128.5) centre (7.3, 128.5) ccw projected
  line L1 (4.75, 42.6) -> (4.75, 128.5) projected
  arc A1 (4.75, 42.6) -> (7.3, 40.05) centre (7.3, 42.6) ccw projected
  line L2 (105.7, 40.05) -> (7.3, 40.05) projected
  arc A2 (105.7, 40.05) -> (108.25, 42.6) centre (105.7, 42.6) ccw projected
  line L3 (108.25, 128.5) -> (108.25, 42.6) projected
  arc A3 (108.25, 128.5) -> (105.7, 131.05) centre (105.7, 128.5) ccw projected
  line L4 (105.7, 131.25) -> (7.3, 131.25)
  arc A4 (7.3, 131.25) -> (4.55, 128.5) centre (7.3, 128.5) ccw
  line L5 (4.55, 128.5) -> (4.55, 42.6)
  arc A5 (4.55, 42.6) -> (7.3, 39.85) centre (7.3, 42.6) ccw
  line L6 (7.3, 39.85) -> (105.7, 39.85)
  arc A6 (105.7, 39.85) -> (108.45, 42.6) centre (105.7, 42.6) ccw
  line L7 (108.45, 42.6) -> (108.45, 128.5)
  arc A7 (108.45, 128.5) -> (105.7, 131.25) centre (105.7, 128.5) ccw
  point P0 (198.3656, 68.5899)
  dimension "d126" = 0.2
  constraints: 8 end point, 8 point on circle, 4 centre point, 7 other
  measures "d126" distance between parallel lines of L0 L4
extrude "Extrusion23" cut sketch "Sketch30" against normal up to surface (6 mm away)
hole "Hole5" at (-89.8656, 63.8221, -12.2578) at (-89.8656, -51.1779, -12.2578) direction (0, 0, -1) diameter 3.4 end up to surface clearance for "Flat Head Machine Screw" size "M3" standard "Ansi Metric M Profile"
hole "Hole6" at (-173.3656, 63.8221, -12.2578) at (-173.3656, -51.1779, -12.2578) direction (0, 0, -1) diameter 3.4 end up to surface clearance for "Flat Head Machine Screw" size "M3" standard "Ansi Metric M Profile"
hole "Hole7" at (-198.3656, 16.8221, -12.2578) at (-198.3656, -4.1779, -12.2578) at (-184.8656, -4.1779, -12.2578) at (-184.8656, 16.8221, -12.2578) direction (0, 0, -1) diameter 2.4 end up to surface clearance for "Flat Head Machine Screw" size "M2" standard "Ansi Metric M Profile"
sketch "Sketch31" plane through (-141.8656, 16.9601, -12.2578) normal (0, 0, 1) x (1, 0, 0)
  line L0 (-27.7565, 64.2739) -> (-27.7565, -85.55) projected
  line L1 (-37.7915, -58.1596) -> (-27.7565, -58.1596)
  line L2 (-27.7565, -58.1596) -> (-27.7565, 42.3788)
  line L3 (-27.7565, 42.3788) -> (-37.7915, 42.3788)
  line L4 (-37.7915, 42.3788) -> (-37.7915, -58.1596)
  point P0 (141.8656, -16.9601)
  constraints: 8 end point, 2 parallel, 1 horizontal, 1 perpendicular, 1 point on line
extrude "Extrusion24" cut sketch "Sketch31" against normal up to surface (5 mm away)
fillet "Fillet1" radius 5 4 edges at (-203.3656, 81.234, -29.7328) (-80.3656, 81.234, -29.7328) (-80.3656, -68.5899, -29.7328) (-203.3656, -68.5899, -29.7328)
body "Solid1"
